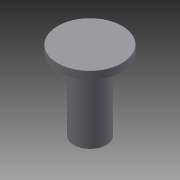
# Autodesk Inventor part: Durometer_Platform
Saved by Autodesk Inventor 2015 (Build 190159000, 159)
## iProperties
Created: 2014-12-16
Part Number: Durometer_Platform
Material: Generic
Document SubType Name: Modeling
Designer: amarschn
Density: 1 g/cm^3
Appearance: Default
Author: amarschn
Autodesk Inventor part; units mm, degrees
ref_plane "YZ Plane" through (0, 0, 0) normal (1, 0, 0) x (0, 1, 0)
ref_plane "XZ Plane" through (0, 0, 0) normal (0, 1, 0) x (-1, 0, 0)
ref_plane "XY Plane" through (0, 0, 0) normal (0, 0, 1) x (1, 0, 0)
sketch "Sketch1" plane through (0, 0, 0) normal (1, 0, 0) x (0, 1, 0)
  line L0 (0, 0) -> (0, -53.8)
  line L1 (0, -53.8) -> (-12.7, -53.8)
  line L2 (-12.7, -53.8) -> (-12.7, -26.9875)
  line L3 (-12.7, -26.9875) -> (-131.6, -26.9875)
  line L4 (-131.6, -26.9875) -> (-131.6, 0)
  line L5 (-131.6, 0) -> (0, 0)
  dimension "d0" = 53.8
  dimension "d1" = 131.6
  dimension "d2" = 26.9875
  dimension "d4" = 12.7
  constraints: 12 end point, 5 perpendicular, 1 vertical
  measures "d0" distance of L0.start L0.end
  measures "d1" distance of L4.end L0.start
  measures "d2" distance of L3.end L4.end
  measures "d4" distance of L0.end L1.end
revolve "Revolution1" add sketch "Sketch1" angle 360 about axis through (0, -131.6, 0) along (0, 1, 0)
chamfer "Chamfer1" distance 0.5 angle 45 1 edges at (0, 0, 53.8)
body "Solid1"
